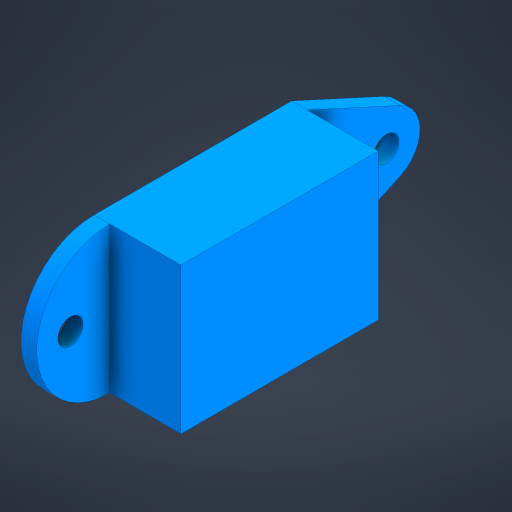
# Autodesk Inventor part: carcasa_giroscopio
Saved by Autodesk Inventor 2023.1 (Build 271208000, 208)
## iProperties
Created: 2022-11-21
Part Number: carcasa_giroscopio
Material: Generic
Document SubType Name: Modeling
Designer: amtat
Density: 1 g/cm^3
Appearance: Default
Author: amtat
Autodesk Inventor part; units mm, degrees
ref_plane "YZ Plane" through (0, 0, 0) normal (1, 0, 0) x (0, 1, 0)
ref_plane "XZ Plane" through (0, 0, 0) normal (0, 1, 0) x (-1, 0, 0)
ref_plane "XY Plane" through (0, 0, 0) normal (0, 0, 1) x (1, 0, 0)
sketch "Sketch1" plane through (0, 0, 0) normal (1, 0, 0) x (0, 1, 0)
  line L0 (0, 0) -> (18.5, 0)
  line L1 (18.5, 0) -> (18.5, -25)
  line L2 (18.5, -25) -> (0, -25)
  line L3 (0, -25) -> (0, 0)
  line L4 (18.5, 0) -> (9.25, 0)
  line L5 (9.25, 0) -> (9.25, 5)
  circle A0 centre (9.25, 5) radius 1.6
  line L6 (9.25, 5) -> (9.25, -35)
  circle A1 centre (9.25, -35) radius 1.6
  arc A2 (18.5, 0) -> (0, 0) centre (9.25, 0) ccw
  line L7 (9.25, -35) -> (9.25, -36.6)
  line L8 (9.25, -36.6) -> (9.25, -39.25)
  arc A3 (5.3854, -36.7685) -> (13.1146, -36.7685) centre (9.25, -35) ccw
  line L9 (0, -25) -> (5.3854, -36.7685)
  line L10 (18.5, -25) -> (13.1146, -36.7685)
  line L11 (18.5, 0) -> (17.5, 0)
  line L12 (17.5, 0) -> (17.5, -24)
  line L13 (17.5, -24) -> (1, -24)
  line L14 (1, -24) -> (1, -1)
  line L15 (1, -1) -> (17.5, -1)
  dimension "d6" = 3.2
  dimension "d0" = 18.5
  dimension "d1" = 25
  dimension "d2" = 9.25
  dimension "d3" = 5
  dimension "d4" = 3.2
  dimension "d5" = 40
  dimension "d7" = 2.65
  dimension "d8" = 1
  dimension "d9" = 24
  dimension "d10" = 16.5
  dimension "d11" = 23
  constraints: 32 end point, 6 perpendicular, 5 point on circle, 4 coincident, 4 point on line, 3 centre point, 2 parallel, 2 tangent, 2 vertical, 1 horizontal, 1 midpoint, 1 vertical alignment, 2 other
  measures "d0" distance of L1.end L2.end
  measures "d1" distance of L0.end L1.end
  measures "d2" distance of L0.end L4.end
  measures "d3" distance of L4.end L5.end
  measures "d4" diameter of A0
  measures "d5" distance of L6.start L6.end
  measures "d7" distance of L7.end L8.end
  measures "d8" distance of L0.end L11.end
  measures "d9" distance of L11.end L12.end
  measures "d10" distance of L12.end L13.end
  measures "d11" distance of L13.end L14.end
extrude "Extrusion1" add sketch "Sketch1" along normal blind 2 contours A2 L0 | L0 L6 L15 L14 L13 L2 L3 | L0 L12 L15 L6 | L2 L6 A1 L8 A3 L9 | L1 L2 L6 L13 L12 L0 | L2 L10 A3 L8 A1 L6
sketch "Sketch2" plane through (2, 0, 0) normal (1, 0, 0) x (0, 0, -1)
  line L0 (36.7685, 13.1146) -> (25, 18.5) projected
  line L1 (25, 18.5) -> (0, 18.5) projected
  arc A0 (0, 18.5) -> (0, 0) centre (0, 9.25) ccw projected
  line L2 (0, 0) -> (25, 0) projected
  line L3 (25, 0) -> (36.7685, 5.3854) projected
  arc A1 (36.7685, 5.3854) -> (36.7685, 13.1146) centre (35, 9.25) ccw projected
  circle A2 centre (35, 9.25) radius 1.6 projected
  circle A3 centre (-5, 9.25) radius 1.6 projected
  line L4 (1, 1) -> (1, 17.5) projected
  line L5 (1, 17.5) -> (24, 17.5) projected
  line L6 (24, 17.5) -> (24, 1) projected
  line L7 (24, 1) -> (1, 1) projected
  line L8 (1, 17.5) -> (24, 17.5) projected
  line L9 (1, 17.5) -> (0, 17.5)
  arc A4 (0, 18.5) -> (0, 0) centre (0, 9.25) ccw projected
  line L10 (0, 17.5) -> (0, 0)
  line L11 (0, 0) -> (25, 0) projected
  line L12 (0, 0) -> (25, 0)
  line L13 (36.7685, 13.1146) -> (25, 18.5) projected
  line L14 (25, 0) -> (25, 18.5)
  line L15 (25, 18.5) -> (0, 18.5) projected
  line L16 (25, 18.5) -> (0, 18.5)
  line L17 (0, 18.5) -> (0, 17.5)
  point P0 (0, 0)
  constraints: 12 end point, 2 collinear, 1 horizontal, 1 parallel, 1 perpendicular, 1 vertical
extrude "Extrusion2" add sketch "Sketch2" along normal blind 6 contours L14 L2 L10 L17 L1
sketch "Sketch4" plane through (8, 0, 0) normal (1, 0, 0) x (0, 0, -1)
  line L0 (0, 0) -> (25, 0) projected
  line L1 (25, 0) -> (25, 18.5) projected
  line L2 (25, 18.5) -> (0, 18.5) projected
  line L3 (0, 18.5) -> (0, 0) projected
  line L4 (1, 17.5) -> (24, 17.5) projected
  line L5 (24, 17.5) -> (24, 1) projected
  line L6 (24, 1) -> (1, 1) projected
  line L7 (1, 1) -> (1, 17.5) projected
  point P0 (0, 0)
extrude "Extrusion4" add sketch "Sketch4" along normal blind 2
sketch "Sketch5" plane through (10, 0, 0) normal (1, 0, 0) x (0, 0, -1)
  line L0 (25, 0) -> (25, 18.5) projected
  line L1 (25, 18.5) -> (0, 18.5) projected
  line L2 (0, 18.5) -> (0, 0) projected
  line L3 (0, 0) -> (25, 0) projected
  line L4 (1, 17.5) -> (24, 17.5) projected
  line L5 (24, 17.5) -> (24, 1) projected
  line L6 (24, 1) -> (1, 1) projected
  line L7 (1, 1) -> (1, 17.5) projected
  point P0 (0, 0)
extrude "Extrusion5" add sketch "Sketch5" along normal blind 1 contours L3 L2 L1 L0 | L4 L5 L6 L7
body "Solid1"
